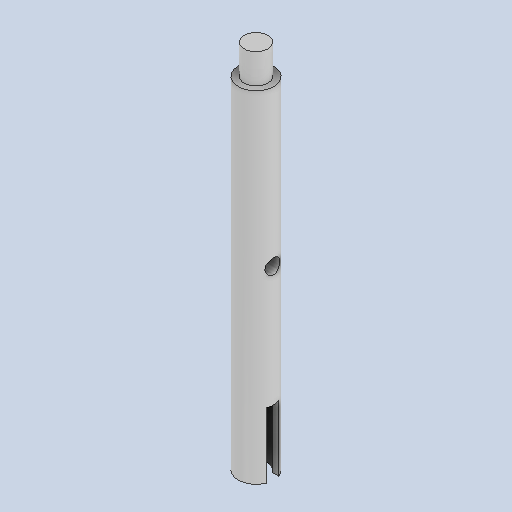
# Autodesk Inventor part: omu_sh_jo_2
Saved by Autodesk Inventor 2025.1 (Build 291241000, 241)
## iProperties
Created: 2024-01-21
Part Number: omu_sh_jo_2
Material: アルミニウム 6061-AHC
Document SubType Name: Modeling
Designer: fhbdh
Density: 2.7 g/cm^3
Appearance: アルミニウム - ダーク
Author: fhbdh
Autodesk Inventor part; units mm, degrees
ref_plane "XZ Plane" through (0, 0, 0) normal (0, 1, 0) x (-1, 0, 0)
ref_plane "XY Plane" through (0, 0, 0) normal (0, 0, 1) x (1, 0, 0)
sketch "スケッチ1" plane through (0, 0, 0) normal (0, 1, 0) x (-1, 0, 0)
  circle A0 centre (0, 0) radius 6
  dimension "d0" = 12
  constraints: 1 centre point, 1 coincident
  measures "d0" diameter of A0
extrude "押し出し1" add sketch "スケッチ1" along normal blind 125
ref_plane "作業平面1" through (6, 0, 0) normal (1, 0, 0) x (0, 1, 0)
sketch "スケッチ2" plane through (6, 0, 0) normal (1, 0, 0) x (0, 1, 0)
  circle A0 centre (62.5, 0) radius 2.5
  line L0 (125, -6) -> (125, 6) projected
  line L1 (125, 0) -> (0, 0) construction
  line L2 (0, -6) -> (0, 6) projected
  dimension "d3" = 5
  dimension "d7" = 62.5
  constraints: 2 end point, 2 midpoint, 1 centre point, 1 horizontal
  measures "d3" diameter of A0
  measures "d7" distance from line of L2 A0.centre
extrude "押し出し2" cut sketch "スケッチ2" against normal through all
sketch "スケッチ3" plane through (0, 125, 0) normal (0, 1, 0) x (1, 0, 0)
  circle A0 centre (0, 0) radius 4
  circle A1 centre (0, 0) radius 6 projected
  dimension "d8" = 8
  constraints: 1 centre point, 1 coincident
  measures "d8" diameter of A0
extrude "押し出し3" cut sketch "スケッチ3" against normal blind 10
sketch "スケッチ4" plane through (0, 0, 0) normal (0, -1, 0) x (1, 0, 0)
  circle A0 centre (0, 0) radius 4
  line L0 (3.4641, 2) -> (5.6569, 2)
  line L1 (3.4641, -2) -> (5.6569, -2)
  circle A1 centre (0, 0) radius 6 projected
  line L2 (0, 0) -> (6, 0) construction
  dimension "d11" = 8
  dimension "d12" = 4
  constraints: 6 end point, 5 point on circle, 2 horizontal, 1 centre point, 1 coincident, 1 parallel, 1 other
  measures "d11" diameter of A0
  measures "d12" distance between parallel lines of L1 L0
extrude "押し出し4" cut sketch "スケッチ4" against normal blind 22 contours A0 | A0 L0 A1 L1 picked at (4.6336, -0.4576)
